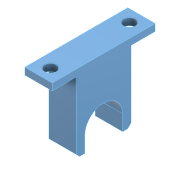
# Autodesk Inventor part: differential stopper
Saved by Autodesk Inventor 2022 (Build 260153000, 153)
## iProperties
Created: 2024-07-09
Part Number: differential stopper
Material: Generic
Document SubType Name: Modeling
Designer: david
Density: 1 g/cm^3
Appearance: Smooth - Dark Forest Green
Author: david
Autodesk Inventor part; units mm, degrees
ref_plane "YZ Plane" through (0, 0, 0) normal (1, 0, 0) x (0, 1, 0)
ref_plane "XZ Plane" through (0, 0, 0) normal (0, 1, 0) x (-1, 0, 0)
ref_plane "XY Plane" through (0, 0, 0) normal (0, 0, 1) x (1, 0, 0)
sketch "Sketch2" plane through (0, 0, 0) normal (1, 0, 0) x (0, 0, -1)
  line L0 (0, 0) -> (0, -18) construction
  line L1 (-8, 0) -> (-8, -18)
  line L2 (8, -18) -> (8, 0)
  arc A0 (8, 0) -> (-8, 0) centre (0, 0) ccw construction
  arc A1 (-8, -18) -> (8, -18) centre (0, -18) ccw construction
  arc A2 (5.5, -18) -> (-5.5, -18) centre (0, -18) ccw
  circle A3 centre (0, -18) radius 4.5 construction
  line L3 (-8, 0) -> (8, 0)
  line L4 (8, -18) -> (5.5, -18)
  arc A4 (-5.5, -18) -> (0, -23.5) centre (0, -18) ccw construction
  arc A5 (0, -23.5) -> (5.5, -18) centre (0, -18) ccw construction
  line L5 (-5.5, -18) -> (-8, -18)
  line L6 (5.5, -18) -> (-5.5, -18) construction
  line L7 (8, -18) -> (5.5, -18)
  line L8 (5.5, -18) -> (5.5, -22.5)
  line L9 (5.5, -22.5) -> (8, -22.5)
  line L10 (8, -22.5) -> (8, -18)
  line L11 (-8, -18) -> (-5.5, -18)
  line L12 (-5.5, -18) -> (-5.5, -22.5)
  line L13 (-5.5, -22.5) -> (-8, -22.5)
  line L14 (-8, -22.5) -> (-8, -18)
  point P0 (0, -9)
  dimension "d2" = 2.5
  dimension "d3" = 9
  dimension "d4" = 1
  dimension "d5" = 18
  dimension "d18" = 4.5
  constraints: 32 end point, 10 point on circle, 6 centre point, 6 perpendicular, 5 parallel, 4 tangent, 3 point on line, 2 coincident, 2 horizontal, 1 collinear, 1 midpoint, 1 vertical
  measures "d2" distance edge to line of A2 L2
  measures "d3" diameter of A3
  measures "d4" radial gap between concentric circles of A2 A3
  measures "d5" distance of L0.start L0.end
  measures "d18" distance of L9.end L2.start
extrude "Extrusion1" add sketch "Sketch2" along normal mid plane 8
sketch "Sketch3" plane through (4, 0, 8) normal (0, 1, 0) x (0, 0, -1)
  line L0 (-7, 0) -> (23, 0)
  line L1 (23, 0) -> (23, 8)
  line L2 (23, 8) -> (-7, 8)
  line L3 (-7, 8) -> (-7, 0)
  line L4 (-7, 0) -> (23, 8) construction
  line L5 (23, 0) -> (-7, 8) construction
  line L6 (0, 8) -> (16, 8) projected
  line L7 (0, 8) -> (0, 0) projected
  point P0 (8, 4)
  dimension "d8" = 7
  constraints: 12 end point, 2 midpoint, 2 parallel, 1 collinear, 1 horizontal, 1 perpendicular
  measures "d8" distance between parallel lines of L7 L3
extrude "Extrusion2" add sketch "Sketch3" against normal blind 2
sketch "Sketch4" plane through (4, -2, 8) normal (0, -1, 0) x (0, 0, -1)
  line L0 (23, 0) -> (23, -8) projected
  line L1 (23, -8) -> (16, -8) projected
  line L2 (16, -8) -> (0, -8) projected
  line L3 (0, -8) -> (0, 0) projected
  line L4 (-7, 0) -> (0, 0) projected
  line L5 (-7, -8) -> (-7, 0) projected
  line L6 (0, -8) -> (-7, -8) projected
  line L7 (16, 0) -> (23, 0) projected
  line L8 (16, 0) -> (16, -8) projected
  line L9 (0, 0) -> (16, 0) projected
  point P0 (19.5, -4)
  point P1 (19.5, -8)
  point P2 (23, -4)
  point P3 (-3.5, -4)
  point P4 (-7, -4)
  point P5 (-3.5, -8)
  constraints: 4 midpoint, 2 horizontal alignment, 2 vertical alignment
hole "Hole1" at (0, -2, -11.5) at (0, -2, 11.5) direction (0, 1, 0) diameter 3.4 end through all
chamfer "Chamfer1" distance 1 angle 45 2 edges at (0, -22.5, -8) (0, -22.5, 8)
equation "\"d18\" = 0.5 * d3"
body "Solid1"
